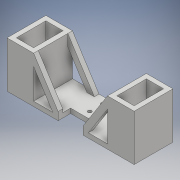
# Autodesk Inventor part: Tablet_joint_Holder
Saved by Autodesk Inventor 2018.3 (Build 223284000, 284)
## iProperties
Created: 2020-10-27
Part Number: Tablet_joint_Holder
Material: Generic
Document SubType Name: Modeling
Designer: chris
Density: 1 g/cm^3
Appearance: Default
Author: chris
Autodesk Inventor part; units mm, degrees
ref_plane "YZ Plane" through (0, 0, 0) normal (1, 0, 0) x (0, 1, 0)
ref_plane "XZ Plane" through (0, 0, 0) normal (0, 1, 0) x (-1, 0, 0)
ref_plane "XY Plane" through (0, 0, 0) normal (0, 0, 1) x (1, 0, 0)
sketch "Sketch6" plane through (0, 0, 0) normal (0, 0, 1) x (1, 0, 0)
  line L0 (40.1, 14.2) -> (56.7, 14.2)
  line L1 (56.7, 14.2) -> (56.7, -14.2)
  line L2 (56.7, -14.2) -> (40.1, -14.2)
  line L3 (40.1, -14.2) -> (40.1, 14.2)
  line L4 (35.6, -18.7) -> (61.2, -18.7)
  line L5 (61.2, -18.7) -> (61.2, 18.7)
  line L6 (61.2, 18.7) -> (35.6, 18.7)
  line L7 (35.6, 18.7) -> (35.6, -18.7)
  line L8 (-40.1, 14.2) -> (-56.7, 14.2)
  line L9 (-56.7, 14.2) -> (-56.7, -14.2)
  line L10 (-56.7, -14.2) -> (-40.1, -14.2)
  line L11 (-40.1, -14.2) -> (-40.1, 14.2)
  line L12 (-35.6, -18.7) -> (-61.2, -18.7)
  line L13 (-61.2, -18.7) -> (-61.2, 18.7)
  line L14 (-61.2, 18.7) -> (-35.6, 18.7)
  line L15 (-35.6, 18.7) -> (-35.6, -18.7)
  point P0 (35.6, 0)
  point P1 (35.6, 0)
  point P2 (-35.6, 0)
  point P3 (-35.6, 0)
  constraints: 32 end point, 4 parallel, 2 perpendicular, 1 horizontal, 1 midpoint, 3 other
extrude "Extrusion4" add sketch "Sketch6" along normal blind 40
sketch "Sketch7" plane through (0, 0, 0) normal (0, 0, -1) x (-1, 0, 0)
  line L0 (-35.6, -18.7) -> (-61.2, -18.7) construction
  line L1 (61.2, 18.7) -> (-61.2, 18.7)
  line L2 (-61.2, 18.7) -> (-61.2, -18.7)
  line L3 (-61.2, -18.7) -> (61.2, -18.7)
  line L4 (61.2, -18.7) -> (61.2, 18.7)
  point P0 (0, 0)
  constraints: 8 end point, 2 parallel, 1 horizontal, 1 perpendicular
extrude "Extrusion5" add sketch "Sketch7" along normal blind 4.5
sketch "Sketch8" plane through (35.6, 18.7, 40) normal (0, 1, 0) x (1, 0, 0)
  line L0 (-71.2, 40) -> (0, 40) construction
  line L1 (0, 40) -> (0, 0) construction
  line L2 (-25.6, 40) -> (0, 0)
  line L3 (0, 11.1306) -> (-18.4764, 40)
  line L4 (-25.6, 40) -> (-18.4764, 40)
  line L5 (0, 11.1306) -> (0, 0)
  point P0 (-35.6, 40)
  constraints: 8 end point, 3 point on line, 1 collinear, 1 other
extrude "Extrusion6" add sketch "Sketch8" against normal blind 4.5
mirror "Mirror3" about plane through (0, 0, 0) normal (0, 1, 0) of "Extrusion6"
mirror "Mirror4" about plane through (0, 0, 0) normal (1, 0, 0) of "Extrusion6", "Mirror3"
sketch "Sketch9" plane through (0, 0, 0) normal (0, 0, 1) x (1, 0, 0)
  line L0 (12, -18.7) -> (12, -6.7)
  line L1 (-12, -6.7) -> (-12, -18.7)
  line L2 (-35.6, -18.7) -> (-10, -18.7) construction
  line L3 (12, -6.7) -> (-12, -6.7)
  line L4 (12, -18.7) -> (-12, -18.7)
  point P0 (0, 0)
  constraints: 8 end point, 1 collinear, 1 horizontal, 1 point on line, 1 vertical
extrude "Extrusion7" cut sketch "Sketch9" along normal mid plane 10
sketch "Sketch10" plane through (0, 0, -4.5) normal (0, 0, -1) x (-1, 0, 0)
  line L0 (12, -6.7) -> (-12, -6.7) construction
  line L1 (10, 18.7) -> (-10, 18.7) construction
  circle A0 centre (0, 12.35) radius 1.8
  circle A1 centre (0, -0.35) radius 1.8
  point P0 (0, 0)
  constraints: 2 centre point
extrude "Extrusion8" cut sketch "Sketch10" against normal blind 10
body "Solid2"
